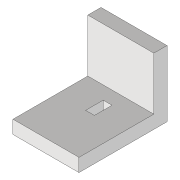
# Autodesk Inventor part: Staender
Saved by Autodesk Inventor 2020 (Build 240168000, 168)
## iProperties
Created: 2020-03-18
Part Number: Staender
Material: Generisch
Document SubType Name: Modeling
Designer: franz
Density: 1 g/cm^3
Appearance: Vorgabe
Author: franz
Autodesk Inventor part; units mm, degrees
ref_plane "YZ Plane" through (0, 0, 0) normal (1, 0, 0) x (0, 1, 0)
ref_plane "XZ Plane" through (0, 0, 0) normal (0, 1, 0) x (-1, 0, 0)
ref_plane "XY Plane" through (0, 0, 0) normal (0, 0, 1) x (1, 0, 0)
sketch "Skizze2" plane through (0, 0, 0) normal (1, 0, 0) x (0, 1, 0)
  line L0 (0, 0) -> (120, 0)
  line L1 (120, 0) -> (120, -30)
  line L2 (120, -30) -> (-30, -30)
  line L3 (-30, -30) -> (-30, 100)
  line L4 (-30, 100) -> (0, 100)
  line L5 (0, 100) -> (0, 0)
  dimension "d0" = 30
  dimension "d1" = 30
  dimension "d2" = 130
  dimension "d3" = 150
  constraints: 12 end point, 5 perpendicular, 1 horizontal
  measures "d0" distance of L3.end L4.end
  measures "d1" distance of L0.end L1.end
  measures "d2" distance of L2.end L3.end
  measures "d3" distance of L1.end L2.end
extrude "Extrusion1" add sketch "Skizze2" along normal blind 150
sketch "Skizze3" plane through (0, -30, -30) normal (0, -1, 0) x (1, 0, 0)
  line L0 (65, 100) -> (85, 100)
  line L1 (85, 100) -> (85, 60)
  line L2 (85, 60) -> (65, 60)
  line L3 (65, 60) -> (65, 100)
  line L4 (150, 130) -> (150, 0) projected
  line L5 (0, 130) -> (0, 0) projected
  line L6 (0, 130) -> (150, 130) projected
  point P0 (0, 30)
  dimension "d6" = 150
  dimension "d7" = 20
  dimension "d8" = 40
  dimension "d9" = 65
  dimension "d10" = 30
  constraints: 8 end point, 2 parallel, 1 horizontal, 1 perpendicular
  measures "d6" distance between parallel lines of L4 L5
  measures "d7" distance of L0.start L0.end
  measures "d8" distance of L2.end L0.start
  measures "d9" distance between parallel lines of L5 L3
  measures "d10" distance between parallel lines of L6 L0
extrude "Extrusion2" cut sketch "Skizze3" against normal through all
equation "\"d1\" = d0"
equation "\"d9\" = -0.5 * d7 + 0.5 * d6"
